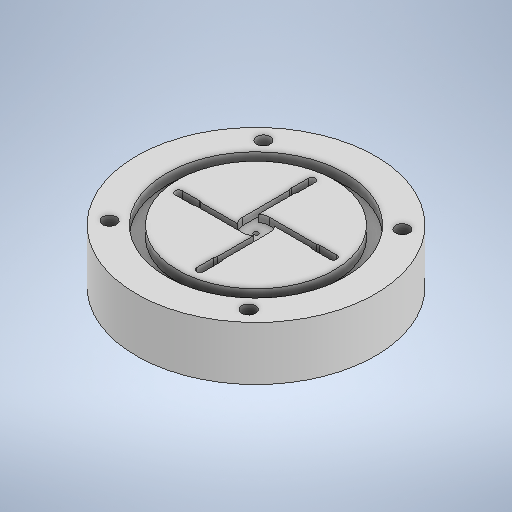
# Autodesk Inventor part: Part6
Saved by Autodesk Inventor 2025 (Build 290162000, 162)
## iProperties
Created: 2026-06-19
Part Number: Part6
Material: Generic
Document SubType Name: Modeling
Designer: saket
Density: 1 g/cm^3
Appearance: Default
Author: saket
Autodesk Inventor part; units mm, degrees
ref_plane "YZ Plane" through (0, 0, 0) normal (1, 0, 0) x (0, 1, 0)
ref_plane "XZ Plane" through (0, 0, 0) normal (0, 1, 0) x (-1, 0, 0)
ref_plane "XY Plane" through (0, 0, 0) normal (0, 0, 1) x (1, 0, 0)
sketch "Sketch1" plane through (0, 0, 0) normal (0, 1, 0) x (-1, 0, 0)
  circle A0 centre (0, 0) radius 0.508
  circle A1 centre (0, 0) radius 3
  line L0 (1.8062, -2.3953) -> (1.8062, -10.5053)
  arc A2 (1.6092, -14.8779) -> (3.197, -14.8779) centre (2.4031, -14.8779) ccw
  line L1 (3.197, -14.8779) -> (3.197, -11.0287)
  line L2 (1.6092, -14.8779) -> (1.6092, -11.0287)
  line L3 (3, 0) -> (3, -10.5053)
  arc A3 (3.197, -11.0287) -> (3, -10.5053) centre (2.4031, -11.0287) ccw
  arc A4 (1.8062, -10.5053) -> (1.6092, -11.0287) centre (2.4031, -11.0287) ccw
  line L4 (0, 3) -> (10.5053, 3)
  line L5 (14.8779, 3.197) -> (11.0287, 3.197)
  line L6 (14.8779, 1.6092) -> (11.0287, 1.6092)
  arc A5 (14.8779, 1.6092) -> (14.8779, 3.197) centre (14.8779, 2.4031) ccw
  arc A6 (11.0287, 3.197) -> (10.5053, 3) centre (11.0287, 2.4031) ccw
  arc A7 (10.5053, 1.8062) -> (11.0287, 1.6092) centre (11.0287, 2.4031) ccw
  line L7 (2.3953, 1.8062) -> (10.5053, 1.8062)
  line L8 (-3, 0) -> (-3, 10.5053)
  line L9 (-3.197, 14.8779) -> (-3.197, 11.0287)
  line L10 (-1.6092, 14.8779) -> (-1.6092, 11.0287)
  arc A8 (-1.6092, 14.8779) -> (-3.197, 14.8779) centre (-2.4031, 14.8779) ccw
  arc A9 (-3.197, 11.0287) -> (-3, 10.5053) centre (-2.4031, 11.0287) ccw
  arc A10 (-1.8062, 10.5053) -> (-1.6092, 11.0287) centre (-2.4031, 11.0287) ccw
  line L11 (-1.8062, 2.3953) -> (-1.8062, 10.5053)
  line L12 (0, -3) -> (-10.5053, -3)
  line L13 (-14.8779, -3.197) -> (-11.0287, -3.197)
  line L14 (-14.8779, -1.6092) -> (-11.0287, -1.6092)
  arc A11 (-14.8779, -1.6092) -> (-14.8779, -3.197) centre (-14.8779, -2.4031) ccw
  arc A12 (-11.0287, -3.197) -> (-10.5053, -3) centre (-11.0287, -2.4031) ccw
  arc A13 (-10.5053, -1.8062) -> (-11.0287, -1.6092) centre (-11.0287, -2.4031) ccw
  line L15 (-2.3953, -1.8062) -> (-10.5053, -1.8062)
  circle A14 centre (0, 0) radius 17.4625
  circle A15 centre (0, 0) radius 20.0025
  circle A16 centre (0, 0) radius 26.67
  line L16 (0, 0) -> (26.67, 0) construction
  circle A17 centre (15.5308, -17.1702) radius 1.524
  circle A18 centre (17.1702, 15.5308) radius 1.524
  circle A19 centre (-15.5308, 17.1702) radius 1.524
  circle A20 centre (-17.1702, -15.5308) radius 1.524
  arc A21 (3.197, -11.0287) -> (1.6092, -11.0287) centre (2.4031, -11.0287) ccw
  arc A22 (11.0287, 3.197) -> (11.0287, 1.6092) centre (11.0287, 2.4031) ccw
  arc A23 (-3.197, 11.0287) -> (-1.6092, 11.0287) centre (-2.4031, 11.0287) ccw
  arc A24 (-11.0287, -3.197) -> (-11.0287, -1.6092) centre (-11.0287, -2.4031) ccw
  line L17 (0, 0) -> (14.8779, 0)
  line L18 (17.0946, 3.5656) -> (17.0946, 3)
  line L19 (17.0946, 1.8062) -> (17.0946, 1.6092)
  point P0 (2.4031, -15.6718)
  dimension "d16" = 34.925
  dimension "d0" = 1.016
  dimension "d1" = 6
  dimension "d13" = 360
  dimension "d17" = 40.005
  dimension "d18" = 53.34
  dimension "d24" = 360
  dimension "d28" = 360
  dimension "d44" = 17.1702
  constraints: 40 end point, 35 point on circle, 24 centre point, 6 coincident, 5 tangent, 4 point on line, 4 vertical, 2 perpendicular, 1 horizontal, 102 other
  measures "d0" diameter of A0
  measures "d1" diameter of A1
  measures "d17" diameter of A15
  measures "d18" diameter of A16
  measures "d44" distance of point (0, 0) L19.end
extrude "Extrusion1" add sketch "Sketch1" along normal blind 12 contours A14 | A16
extrude "Extrusion2" add sketch "Sketch1" along normal blind 10.3632 contours A1 | L3 A21 L0 A1 | A1 L4 A22 L7 | A3 L1 A2 L2 A4 A21 | A22 A6 L5 A5 L6 A7 | L12 A24 L15 A1 | A1 L8 A23 L11 | A12 L13 A11 L14 A13 A24 | A23 A9 L9 A8 L10 A10
extrude "Extrusion3" add sketch "Sketch1" along normal blind 9.6215 contours A15
thread "Thread1" size "M3x0.5" class "6H" standard "ANSI Metric M Profile" length 10
thread "Thread2" size "M3x0.5" class "6H" standard "ANSI Metric M Profile" length 10
thread "Thread3" size "M3x0.5" class "6H" standard "ANSI Metric M Profile" length 10
thread "Thread4" size "M3x0.5" class "6H" standard "ANSI Metric M Profile" length 10
sketch "Sketch2" plane through (0, 0, 0) normal (0, -1, 0) x (1, 0, 0)
  circle A0 centre (0, 0) radius 4
  circle A1 centre (0, 0) radius 0.508 projected
  circle A2 centre (0, 0) radius 5
  dimension "d46" = 8
  dimension "d47" = 10
  constraints: 2 centre point, 2 coincident
  measures "d46" diameter of A0
  measures "d47" diameter of A2
extrude "Extrusion4" cut sketch "Sketch2" against normal blind 4 contours A2
thread "Thread5" size "M8x1.25" class "6g" standard "ANSI Metric M Profile" length 10
body "Solid1"
